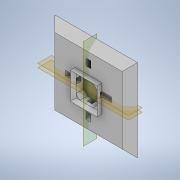
# Autodesk Inventor part: clear-square-reed-2
Saved by Autodesk Inventor 2021 (Build 250183000, 183)
## iProperties
Created: 2020-12-08
Part Number: clear-square-reed-2
Material: Generic
Document SubType Name: Modeling
Designer: Luke Kamols
Density: 1 g/cm^3
Appearance: Default
Author: Luke Kamols
Autodesk Inventor part; units mm, degrees
ref_plane "YZ Plane" through (0, 0, 0) normal (1, 0, 0) x (0, 1, 0)
ref_plane "XZ Plane" through (0, 0, 0) normal (0, 1, 0) x (-1, 0, 0)
sketch "Sketch1" plane through (0, 0, 0) normal (0, 0, 1) x (1, 0, 0)
  line L0 (0, 0) -> (44, 0)
  line L1 (44, 0) -> (44, 44)
  line L2 (44, 44) -> (0, 44)
  line L3 (0, 44) -> (0, 0)
  line L4 (0, 0) -> (0.5, 0)
  line L5 (0.5, 0) -> (0.5, 0.5)
  line L6 (0.5, 0.5) -> (43.5, 0.5)
  line L7 (43.5, 0.5) -> (43.5, 43.5)
  line L8 (43.5, 43.5) -> (0.5, 43.5)
  line L9 (0.5, 43.5) -> (0.5, 0.5)
  dimension "d0" = 44
  dimension "d1" = 44
  dimension "d103" = 0.5
  dimension "d104" = 0.5
  dimension "d105" = 43
  dimension "d106" = 43
  constraints: 20 end point, 4 parallel, 3 perpendicular, 2 horizontal, 1 point on line
  measures "d0" distance of L2.end L1.end
  measures "d1" distance of L1.end L0.end
  measures "d103" distance of L0.start L4.end
  measures "d104" distance of L4.end L5.end
  measures "d105" distance of L8.end L7.end
  measures "d106" distance of L7.end L6.end
extrude "Extrusion1" add sketch "Sketch1" along normal blind 4 contours L9 L8 L7 L6
chamfer "Chamfer1" distance 4 angle 45 4 edges at (43.5, 22, 4) (22, 0.5, 4) (0.5, 22, 4) (22, 43.5, 4)
sketch "Sketch2" plane through (0, 0, 4) normal (0, 0, 1) x (1, 0, 0)
  line L0 (4, 4) -> (40, 40)
  line L1 (22, 16.5) -> (16.5, 16.5)
  line L2 (16.5, 16.5) -> (16.5, 27.5)
  line L3 (16.5, 27.5) -> (27.5, 27.5)
  line L4 (27.5, 27.5) -> (27.5, 16.5)
  line L5 (27.5, 16.5) -> (22, 16.5)
  line L6 (27.5, 27.5) -> (27.5, 25.5)
  arc A0 (18.5, 27.5) -> (16.5, 25.5) centre (18.5, 25.5) ccw
  line L7 (18.5, 25.5) -> (18.5, 18.5)
  line L8 (18.5, 18.5) -> (25.5, 18.5)
  line L9 (25.5, 18.5) -> (25.5, 25.5)
  arc A1 (16.5, 18.5) -> (18.5, 16.5) centre (18.5, 18.5) ccw
  arc A2 (25.5, 16.5) -> (27.5, 18.5) centre (25.5, 18.5) ccw
  arc A3 (27.5, 25.5) -> (25.5, 27.5) centre (25.5, 25.5) ccw
  line L10 (27.5, 18.5) -> (25.5, 16.5)
  line L11 (18.5, 16.5) -> (16.5, 18.5)
  line L12 (16.5, 25.5) -> (18.5, 27.5)
  line L13 (25.5, 27.5) -> (27.5, 25.5)
  point P0 (0, 0)
  dimension "d86" = 2
  constraints: 28 end point, 13 point on line, 8 point on circle, 4 centre point, 4 tangent, 3 coincident, 3 perpendicular
  measures "d86" distance of L6.end L3.end
extrude "Extrusion2" cut sketch "Sketch2" against normal blind 3 contours L0 L11 L2 L12 L3 L13 | L8 L9 L0 L13 L4 L10 L5 L1 L11 | L0 L9 L8
ref_plane "Work Plane4" through (27.5, 27.5, 4) normal (0.7071, -0.7071, 0) x (0, 0, 1)
sketch "Sketch15" plane through (0, 0, 4) normal (0, 0, 1) x (1, 0, 0)
  line L0 (18.5, 16.5) -> (16.5, 18.5) projected
  line L1 (16.5, 18.5) -> (16.5, 25.5) projected
  line L2 (16.5, 25.5) -> (18.5, 27.5) projected
  line L3 (18.5, 27.5) -> (25.5, 27.5) projected
  line L4 (25.5, 27.5) -> (27.5, 25.5) projected
  line L5 (27.5, 25.5) -> (27.5, 18.5) projected
  line L6 (27.5, 18.5) -> (25.5, 16.5) projected
  line L7 (25.5, 16.5) -> (18.5, 16.5) projected
  line L8 (16.5, 18.5) -> (16.5, 25.5) projected
  line L9 (15, 22.9038) -> (15, 29)
  line L10 (15, 29) -> (29, 29)
  line L11 (29, 29) -> (29, 15)
  line L12 (29, 15) -> (15, 15)
  line L13 (15, 15) -> (15, 29)
  line L14 (16.5, 18.5) -> (16.5, 16.5)
  line L15 (16.5, 16.5) -> (18.5, 16.5)
  line L16 (25.5, 16.5) -> (27.5, 16.5)
  line L17 (27.5, 16.5) -> (27.5, 18.5)
  line L18 (27.5, 25.5) -> (27.5, 27.5)
  line L19 (25.5, 27.5) -> (27.5, 25.5) projected
  line L20 (27.5, 27.5) -> (25.5, 27.5)
  line L21 (18.5, 27.5) -> (16.5, 27.5)
  line L22 (16.5, 27.5) -> (16.5, 25.5)
  point P0 (0, 0)
  constraints: 26 end point, 6 perpendicular, 5 point on line, 2 vertical, 1 horizontal
extrude "Extrusion7" add sketch "Sketch15" along normal blind 2.5
chamfer "Chamfer6" distance 1.5 angle 45 4 edges at (22, 16.5, 6.5) (16.5, 22, 6.5) (27.5, 22, 6.5) (22, 27.5, 6.5)
sketch "Sketch16" plane through (0, 0, 4) normal (0, 0, 1) x (1, 0, 0)
  line L0 (16.5, 18.5) -> (16.5, 16.5) projected
  line L1 (16.5, 16.5) -> (18.5, 16.5) projected
  line L2 (18.5, 16.5) -> (16.5, 18.5) projected
  line L3 (27.5, 16.5) -> (27.5, 18.5) projected
  line L4 (27.5, 18.5) -> (25.5, 16.5) projected
  line L5 (25.5, 16.5) -> (27.5, 16.5) projected
  line L6 (25.5, 27.5) -> (27.5, 25.5) projected
  line L7 (27.5, 27.5) -> (25.5, 27.5) projected
  line L8 (25.5, 27.5) -> (27.5, 25.5) projected
  line L9 (27.5, 25.5) -> (27.5, 27.5) projected
  line L10 (18.5, 27.5) -> (16.5, 27.5) projected
  line L11 (16.5, 27.5) -> (16.5, 25.5) projected
  line L12 (16.5, 25.5) -> (18.5, 27.5) projected
  point P0 (0, 0)
extrude "Extrusion8" add sketch "Sketch16" along normal blind 1
ref_plane "Work Plane6" through (22, 18.5, 1) normal (-1, 0, 0) x (0, 0, 1)
ref_plane "Work Plane7" through (18.5, 22, 1) normal (0, 1, 0) x (1, 0, 0)
sketch "Sketch17" plane through (18.5, 22, 1) normal (0, 1, 0) x (1, 0, 0)
  line L0 (7, -4) -> (7, 0) projected
  line L1 (7, 0) -> (0, 0) projected
  line L2 (0, -4) -> (0, 0) projected
  line L3 (7, -4) -> (0, -4) projected
  line L4 (3.5, 0) -> (2.25, 0)
  line L5 (2.25, 0) -> (2.25, -2.5)
  line L6 (2.25, -2.5) -> (4.75, -2.5)
  line L7 (4.75, -2.5) -> (4.75, 0)
  point P0 (-18.5, 1)
  dimension "d109" = 1.25
  dimension "d110" = 2.5
  dimension "d111" = 2.5
  constraints: 8 end point, 3 perpendicular, 2 point on line, 1 midpoint
  measures "d109" distance of L4.start L4.end
  measures "d110" distance of L4.end L5.end
  measures "d111" distance of L5.end L6.end
sketch "Sketch18" plane through (22, 18.5, 1) normal (-1, 0, 0) x (0, 0, 1)
  line L0 (4, 7) -> (0, 7) projected
  line L1 (0, 7) -> (0, 0) projected
  line L2 (4, 0) -> (0, 0) projected
  line L3 (4, 7) -> (4, 0) projected
  line L4 (0, 3.5) -> (1.25, 3.5)
  line L5 (1.25, 3.5) -> (1.25, -6.5)
  line L6 (1.25, -6.5) -> (6.9224, -12.1724)
  line L7 (1.25, 3.5) -> (1.25, 4.137)
  line L8 (1.25, 4.137) -> (1.25, 14.137)
  line L9 (1.25, 14.137) -> (10.5582, 23.4452)
  point P0 (-1, -18.5)
  dimension "d113" = 10
  dimension "d114" = 135
  constraints: 12 end point, 1 horizontal, 1 midpoint, 1 perpendicular, 1 point on line
  measures "d113" distance of L4.end L5.end
  measures "d114" angle of L6 L5
sweep "Sweep4" cut profiles "Sketch17" path "Sketch18" path curves L5 L6 contours L7 L6 L5 L1
sweep "Sweep5" cut profiles "Sketch17" path "Sketch18" path curves L7 L8 L9 contours L7 L6 L5 L1
ref_plane "Work Plane8" through (18.5, 24, 1) normal (0, 1, 0) x (1, 0, 0)
sketch "Sketch19" plane through (22, 18.5, 1) normal (-1, 0, 0) x (0, 0, 1)
  line L0 (-2.3, 5.5) -> (6.8, 5.5) projected
  line L1 (4, 7) -> (0, 7) projected
  line L2 (0, 7) -> (0, 0) projected
  line L3 (4, 0) -> (0, 0) projected
  line L4 (4, 7) -> (4, 0) projected
  line L5 (4, 0) -> (4, 7) projected
  line L6 (4, 5.5) -> (4, 4.25)
  line L7 (4, 4.25) -> (1.5, 4.25)
  line L8 (1.5, 4.25) -> (1.5, 6.75)
  line L9 (1.5, 6.75) -> (4, 6.75)
  line L10 (4, 6.75) -> (4, 4.25)
  point P0 (-1, -18.5)
  dimension "d127" = 1.25
  dimension "d128" = 2.5
  dimension "d129" = 2.5
  constraints: 10 end point, 3 point on line, 2 parallel, 1 horizontal, 1 perpendicular
  measures "d127" distance of L6.start L6.end
  measures "d128" distance of L8.end L9.end
  measures "d129" distance of L7.end L8.end
sketch "Sketch20" plane through (18.5, 24, 1) normal (0, 1, 0) x (1, 0, 0)
  line L0 (3.5, 2.3) -> (3.5, -6.8) projected
  line L1 (3.5, -4) -> (3.5, -2.75)
  line L2 (3.5, -2.75) -> (-6.5, -2.75)
  line L3 (-6.5, -2.75) -> (-11.0554, -7.3054)
  line L4 (3.5, -2.75) -> (13.5, -2.75)
  line L5 (13.5, -2.75) -> (17.1075, -6.3575)
  point P0 (-18.5, 1)
  point P1 (3.5, -4)
  dimension "d130" = 1.25
  dimension "d131" = 10
  dimension "d132" = 135
  dimension "d134" = 10
  constraints: 10 end point, 2 perpendicular, 1 point on line
  measures "d130" distance of L1.start L1.end
  measures "d131" distance of L1.end L2.end
  measures "d132" angle of L3 L2
  measures "d134" distance of L1.end L4.end
sweep "Sweep6" cut profiles "Sketch19" path "Sketch20" path curves L5 L4 L2 L3 contours L8 L9 L4 L0 | L0 L4 L7 L8
body "Solid1"
